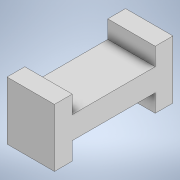
# Autodesk Inventor part: cable_jig_lock
Saved by Autodesk Inventor 2022 (Build 260153000, 153)
## iProperties
Created: 2022-03-09
Part Number: cable_jig_lock
Material: Generic
Document SubType Name: Modeling
Designer: kylem
Density: 1 g/cm^3
Appearance: Default
Author: kylem
Autodesk Inventor part; units mm, degrees
ref_plane "YZ Plane" through (0, 0, 0) normal (1, 0, 0) x (0, 1, 0)
ref_plane "XZ Plane" through (0, 0, 0) normal (0, 1, 0) x (-1, 0, 0)
ref_plane "XY Plane" through (0, 0, 0) normal (0, 0, 1) x (1, 0, 0)
sketch "Sketch1" plane through (0, 0, 0) normal (0, 1, 0) x (-1, 0, 0)
  line L0 (0, 0) -> (8, 0)
  line L1 (8, 0) -> (8, -20)
  line L2 (8, -20) -> (0, -20)
  line L3 (0, -20) -> (0, 0)
  dimension "d0" = 8
  dimension "d1" = 20
  constraints: 8 end point, 2 parallel, 1 horizontal, 1 perpendicular
  measures "d0" distance of L1.end L2.end
  measures "d1" distance of L0.end L1.end
extrude "Extrusion1" add sketch "Sketch1" along normal blind 3.8
sketch "Sketch2" plane through (0, 0, 0) normal (1, 0, 0) x (0, 0, -1)
  line L0 (20, 3.8) -> (0, 3.8) projected
  line L1 (0, 3.8) -> (0, 6.8)
  line L2 (0, 6.8) -> (3, 6.8)
  line L3 (3, 6.8) -> (3, -3)
  line L4 (3, -3) -> (0, -3)
  line L5 (0, -3) -> (0, 6.8)
  line L6 (0, 3.8) -> (20, 3.8)
  line L7 (10, 3.8) -> (10, 4.6084)
  line L8 (20, 6.8) -> (17, 6.8)
  line L9 (17, 6.8) -> (17, -3)
  line L10 (17, -3) -> (20, -3)
  line L11 (20, -3) -> (20, 6.8)
  point P0 (0, 0)
  point P1 (0, 3.8)
  dimension "d4" = 3
  dimension "d5" = 3
  dimension "d6" = 9.8
  constraints: 22 end point, 4 symmetric about line, 2 parallel, 2 vertical, 1 horizontal, 1 midpoint, 1 perpendicular
  measures "d4" distance of L0.end L1.end
  measures "d5" distance of L3.end L4.end
  measures "d6" distance of L2.end L3.end
extrude "Extrusion2" add sketch "Sketch2" against normal blind 8
body "Solid1"
